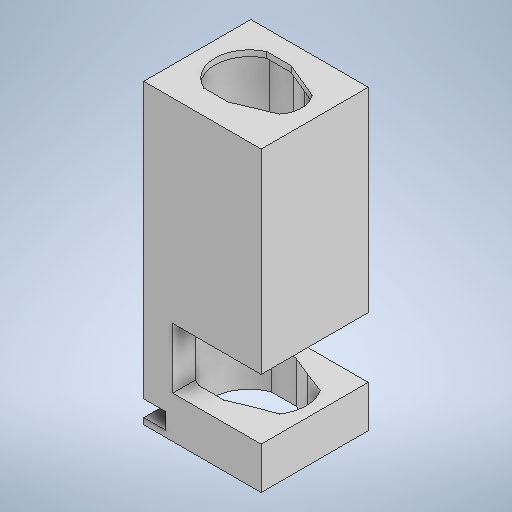
# Autodesk Inventor part: PipetteSleeve
Saved by Autodesk Inventor 2025.1 (Build 291241000, 241)
## iProperties
Created: 2025-01-27
Part Number: PipetteSleeve
Material: Generic
Document SubType Name: Modeling
Designer: 13156
Density: 1 g/cm^3
Appearance: Default
Author: 13156
Autodesk Inventor part; units mm, degrees
ref_plane "YZ Plane" through (0, 0, 0) normal (1, 0, 0) x (0, 1, 0)
ref_plane "XZ Plane" through (0, 0, 0) normal (0, 1, 0) x (-1, 0, 0)
ref_plane "XY Plane" through (0, 0, 0) normal (0, 0, 1) x (1, 0, 0)
sketch "Sketch1" plane through (0, 0, 0) normal (0, 1, 0) x (-1, 0, 0)
  arc A0 (8.935, -11.5681) -> (8.935, 13.2319) centre (3.9712, 0.8319) ccw
  line L0 (8.935, 13.2319) -> (0.335, 13.2319)
  line L1 (8.935, -11.5681) -> (0.335, -11.5681)
  line L2 (0.335, 13.2319) -> (-6.2216, 10.5319)
  line L3 (0.335, -11.5681) -> (-6.2216, -8.8681)
  line L4 (-6.2216, 10.5319) -> (-13.3216, 7.8319)
  line L5 (-6.2216, -8.8681) -> (-13.3216, -6.1681)
  arc A1 (-13.3216, 7.8319) -> (-13.3216, -6.1681) centre (-3.005, 0.8319) ccw
  line L6 (21.9588, 18.8319) -> (-18.0412, 18.8319)
  line L7 (-18.0412, 18.8319) -> (-18.0412, -17.1681)
  line L8 (-18.0412, -17.1681) -> (21.9588, -17.1681)
  line L9 (21.9588, -17.1681) -> (21.9588, 18.8319)
  line L10 (8.935, -11.5681) -> (8.935, 13.2319) construction
  line L11 (-15.9151, 0.8319) -> (22.2552, 0.8319) construction
  line L12 (0.335, -11.5681) -> (0.335, 13.2319) construction
  line L13 (-13.3216, -6.1681) -> (-13.3216, 8.7819) construction
  point P0 (0, 0)
  point P1 (17.3278, 0.8319)
  point P2 (-15.4722, 0.8319)
  point P3 (4.635, -11.5681)
  point P4 (-18.0412, 0.8319)
  point P5 (3.1701, 0.8319)
  dimension "d13" = 36
  dimension "d14" = 40
  dimension "d15" = 32.8
  dimension "d82" = 24.8
  dimension "d83" = 14
  dimension "d84" = 7.1
  dimension "d85" = 6.5566
  dimension "d86" = 2.7
  dimension "d87" = 13.3566
  dimension "d88" = 12.4672
  dimension "d89" = 2.569
  dimension "d90" = 24.8
  dimension "d92" = 3.1701
  dimension "d93" = 0.8319
  dimension "d94" = 0.335
  constraints: 28 end point, 6 point on circle, 4 horizontal, 3 equal length, 3 midpoint, 2 centre point, 2 parallel, 1 perpendicular, 1 point on line, 1 vertical, 4 other
  measures "d13" distance of L6.end L7.end
  measures "d14" distance of L7.end L8.end
  measures "d15" distance of point (-15.472, 0.832) point (17.328, 0.832)
  measures "d82" distance from line of L0 point (4.635, -11.568)
  measures "d83" distance of L4.end L5.end
  measures "d84" horizontal distance of L3.end L5.end
  measures "d85" horizontal distance of L1.end L3.end
  measures "d86" vertical distance of L1.end L3.end
  measures "d87" radius of A0
  measures "d88" radius of A1
  measures "d89" distance of point (-18.041, 0.832) point (-15.472, 0.832)
  measures "d90" distance of L10.end L1.start
  measures "d92" horizontal distance of point (0, 0) point (3.17, 0.832)
  measures "d93" vertical distance of point (0, 0) point (3.17, 0.832)
  measures "d94" distance from line of point (0, 0) L12
extrude "Extrusion1" add sketch "Sketch1" along normal blind 104.4 draft 0.5
sketch "Sketch2" plane through (0, 0, 0) normal (0, -1, 0) x (1, 0, 0)
  line L0 (-21.9588, -17.1681) -> (-21.9588, 18.8319) projected
  line L1 (18.0412, -17.1681) -> (-21.9588, -17.1681) projected
  line L2 (-21.9588, 18.8319) -> (18.0412, 18.8319)
  line L3 (18.0412, 18.8319) -> (18.0412, -17.1681)
  line L4 (18.0412, -17.1681) -> (-21.9588, -17.1681)
  line L5 (-21.9588, -17.1681) -> (-21.9588, 18.8319)
  line L6 (-21.9588, 18.8319) -> (-22.8699, 19.743) projected
  line L7 (18.9523, -18.0792) -> (18.9523, 19.743) projected
  line L8 (-22.8699, 19.743) -> (18.9523, 19.743)
  line L9 (18.9523, 19.743) -> (18.9523, -18.0792)
  line L10 (18.9523, -18.0792) -> (-22.8699, -18.0792)
  line L11 (-22.8699, -18.0792) -> (-22.8699, 19.743)
  point P0 (0, 0)
  point P1 (18.9523, 19.743)
  constraints: 16 end point, 4 parallel, 2 horizontal, 2 perpendicular
extrude "Extrusion2" add sketch "Sketch2" against normal blind 104.4
sketch "Sketch3" plane through (18.9523, 0, 19.743) normal (1, 0, 0) x (0, 0, -1)
  line L0 (42, 38.2) -> (-1, 38.2)
  line L1 (-1, 38.2) -> (-1, 17.7)
  line L2 (-1, 17.7) -> (42, 17.7)
  line L3 (42, 17.7) -> (42, 38.2)
  line L4 (37.8222, 104.4) -> (0, 104.4) projected
  line L5 (0, 0) -> (0, 104.4) projected
  point P0 (19.743, 0)
  point P1 (17.836, -13.8464)
  point P2 (-1, 27.95)
  point P3 (0, 38.2)
  point P4 (0, 17.7)
  dimension "d21" = 20.5
  dimension "d23" = 43
  dimension "d25" = 86.7
  dimension "d26" = 1
  constraints: 8 end point, 2 parallel, 1 horizontal, 1 midpoint, 1 perpendicular
  measures "d21" distance of L2.end L0.start
  measures "d23" distance from line of L1.end L3
  measures "d25" distance between parallel lines of L4 L2
  measures "d26" distance from line of L5 point (-1, 27.95)
extrude "Extrusion3" cut sketch "Sketch3" against normal blind 30 contours L3 L2 L5 L0
sketch "Sketch5" plane through (0, 104.4, 0) normal (0, 1, 0) x (1, 0, 0)
  line L0 (-8.7562, 10.657) -> (-0.5153, 10.657) construction
  line L1 (-8.7562, 10.657) -> (-8.7562, -13.1004) construction
  line L2 (-0.5153, 10.657) -> (-0.5153, -15.3944) construction
  line L3 (5.8861, 8.0209) -> (12.7234, 5.4208) construction
  line L4 (12.7234, 5.4208) -> (12.7234, -11.6107) construction
  line L5 (-21.2529, -0.8319) -> (27.3755, -0.8319) construction
  line L6 (-8.7562, 9.857) -> (-0.5153, 9.857)
  line L7 (-0.5153, 9.857) -> (11.7259, 4.7413)
  arc A0 (11.7259, -6.4051) -> (11.7259, 4.7413) centre (5.1127, -0.8319) ccw
  line L8 (11.7259, -6.4051) -> (-0.5153, -11.5208)
  line L9 (-0.5153, -11.5208) -> (-8.7562, -11.5208)
  arc A1 (-8.7562, 9.857) -> (-8.7562, -11.5208) centre (-3.8596, -0.8319) ccw
  line L10 (-0.5153, 10.657) -> (5.8861, 8.0209) projected
  line L11 (-0.5153, -12.3208) -> (-8.7562, -12.3208) projected
  arc A2 (12.7234, -7.0846) -> (12.7234, 5.4208) centre (3.005, -0.8319) ccw projected
  line L12 (-22.8699, 18.0792) -> (18.9523, 18.0792) projected
  line L13 (18.9523, -19.743) -> (-22.8699, -19.743) projected
  line L14 (-22.8699, 18.0792) -> (18.9523, 18.0792)
  line L15 (18.9523, 18.0792) -> (18.9523, -19.743)
  line L16 (18.9523, -19.743) -> (-22.8699, -19.743)
  line L17 (-22.8699, -19.743) -> (-22.8699, 18.0792)
  arc A3 (-8.7562, 10.657) -> (-8.7562, -12.3208) centre (-3.9712, -0.8319) ccw projected
  point P0 (0, 0)
  point P1 (-4.6357, 9.857)
  point P2 (-4.6357, -12.3208)
  point P3 (13.7611, -0.8319)
  point P4 (14.5611, -0.8319)
  point P5 (18.9523, 18.0792)
  point P6 (-22.8699, -19.743)
  point P7 (-16.4167, -0.8319)
  point P8 (-15.6167, -0.8319)
  dimension "d46" = 0.299
  dimension "d47" = 0.8
  dimension "d48" = 0.8
  dimension "d51" = 8.6484
  dimension "d52" = 0.8
  dimension "d95" = 0.8
  constraints: 24 end point, 8 point on circle, 4 point on line, 3 perpendicular, 3 vertical, 2 centre point, 2 horizontal, 2 midpoint, 2 parallel, 1 equal length, 1 other
  measures "d46" angle of L10 L7
  measures "d47" distance from line of L0 point (-4.636, 9.857)
  measures "d48" distance from line of point (-4.636, -12.321) L9
  measures "d51" radius of A0
  measures "d52" distance of point (14.561, -0.832) point (13.761, -0.832)
  measures "d95" distance of point (-16.417, -0.832) point (-15.617, -0.832)
extrude "Extrusion4" add sketch "Sketch5" against normal blind 2
sketch "Sketch6" plane through (-22.8699, 0, -18.0792) normal (-1, 0, 0) x (0, 0, 1)
  line L0 (37.8222, 5.6) -> (0, 5.6)
  line L1 (0, 5.6) -> (0, 11.1)
  line L2 (0, 11.1) -> (37.8222, 11.1)
  line L3 (37.8222, 11.1) -> (37.8222, 5.6)
  line L4 (37.8222, 0) -> (37.8222, 104.4) projected
  line L5 (0, 0) -> (0, 104.4) projected
  line L6 (37.8222, 0) -> (0, 0) projected
  point P0 (18.0792, 0)
  point P1 (37.8222, 8.35)
  point P2 (0, 5.6)
  dimension "d55" = 5.5
  dimension "d56" = 0
  dimension "d57" = 0
  dimension "d58" = 5.6
  constraints: 8 end point, 2 parallel, 1 horizontal, 1 midpoint, 1 perpendicular
  measures "d55" distance between parallel lines of L2 L0
  measures "d56" distance from line of L4 point (37.822, 8.35)
  measures "d57" distance between parallel lines of L5 L1
  measures "d58" distance between parallel lines of L0 L6
extrude "Extrusion5" cut sketch "Sketch6" against normal blind 4.5 contours L0 L1 L2 L3
sketch "Sketch7" plane through (-18.3699, 0, -18.0792) normal (-1, 0, 0) x (0, 0, 1)
  line L0 (0, 0) -> (0, 17.7) projected
  line L1 (0, 11.1) -> (37.8222, 11.1) projected
  line L2 (0, 5.6) -> (4, 5.6)
  line L3 (4, 5.6) -> (4, 11.1)
  line L4 (4, 11.1) -> (0, 11.1)
  line L5 (0, 11.1) -> (0, 5.6)
  line L6 (37.8222, 5.6) -> (0, 5.6) projected
  point P0 (18.0792, 0)
  dimension "d61" = 4
  dimension "d108" = 0
  constraints: 8 end point, 2 parallel, 2 point on line, 1 horizontal, 1 perpendicular
  measures "d61" distance between parallel lines of L0 L3
  measures "d108" distance between parallel lines of L6 L2
extrude "Extrusion6" cut sketch "Sketch7" against normal blind 10.5
sketch "Sketch8" plane through (0, 0, 0) normal (0, -1, 0) x (1, 0, 0)
  line L0 (-20.8699, -16.5792) -> (19.1301, -16.5792)
  line L1 (19.1301, -16.5792) -> (19.1301, 19.9208)
  line L2 (19.1301, 19.9208) -> (-20.8699, 19.9208)
  line L3 (-20.8699, 19.9208) -> (-20.8699, -16.5792)
  line L4 (-22.8699, -18.0792) -> (18.9523, -18.0792) projected
  line L5 (-22.8699, 19.743) -> (-22.8699, -18.0792) projected
  line L6 (-22.8699, 19.743) -> (-22.8699, -18.0792) projected
  line L7 (18.9523, -18.0792) -> (18.9523, 19.743) projected
  line L8 (-22.8699, -18.0792) -> (18.9523, -18.0792)
  line L9 (18.9523, -18.0792) -> (18.9523, 19.743)
  line L10 (18.9523, 19.743) -> (-22.8699, 19.743)
  line L11 (-22.8699, 19.743) -> (-22.8699, -18.0792)
  point P0 (0, 0)
  dimension "d68" = 36.5
  dimension "d69" = 40
  dimension "d70" = 1.5
  dimension "d71" = 2
  constraints: 16 end point, 4 parallel, 2 horizontal, 2 perpendicular
  measures "d68" distance of L2.end L0.start
  measures "d69" distance of L0.start L0.end
  measures "d70" distance between parallel lines of L4 L0
  measures "d71" distance between parallel lines of L5 L3
extrude "Extrusion7" cut sketch "Sketch8" against normal blind 126.8375 contours L0 L7 L4 L5 L10 L3
sketch "Sketch9" plane through (-20.8699, 11.1, -16.5792) normal (-1, 0, 0) x (0, 0, 1)
  circle A0 centre (16.5792, 23.9) radius 1.95
  circle A1 centre (16.5792, 58.3) radius 1.95
  line L0 (16.5792, -11.1) -> (16.5792, 93.3) construction
  line L1 (11.8379, 93.3) -> (22.9843, 93.3) construction
  line L2 (0, 93.3) -> (36.3222, 93.3) projected
  line L3 (36.3222, -11.1) -> (0, -11.1) projected
  point P0 (36.5, 93.4)
  point P1 (36.5, -11)
  point P2 (0, -11.1)
  dimension "d74" = 3.9
  dimension "d75" = 0
  dimension "d76" = 0
  dimension "d78" = 35
  dimension "d79" = 35
  constraints: 2 centre point, 2 end point, 1 equal radius, 1 point on line, 1 vertical, 2 other
  measures "d74" diameter of A0
  measures "d75" distance from line of L0 A0.centre
  measures "d76" distance from line of L0 A1.centre
extrude "Extrusion8" cut sketch "Sketch9" against normal blind 14.025
sketch "Sketch11" plane through (-11.0477, 17.7, 19.743) normal (0, 0, 1) x (1, 0, 0)
  line L0 (30, -17.7) -> (30, 0) projected
  line L1 (-9.8222, -12.1) -> (-9.8222, -17.7) projected
  line L2 (30, -17.7) -> (-9.8222, -17.7)
  line L3 (-9.8222, -17.7) -> (-9.8222, -14.2)
  line L4 (-9.8222, -14.2) -> (30, -14.2)
  line L5 (30, -14.2) -> (30, -17.7)
  point P0 (11.0477, -17.7)
  dimension "d102" = 3.5
  constraints: 8 end point, 2 parallel, 1 horizontal, 1 perpendicular, 1 point on line
  measures "d102" distance between parallel lines of L2 L4
extrude "Extrusion10" cut sketch "Sketch11" against normal blind 136.15
chamfer "Chamfer1" distance 5 angle 45 1 edges at (-18.3699, 8.35, 19.743)
body "Solid1"
